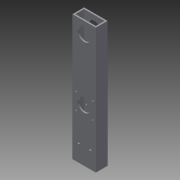
# Autodesk Inventor part: ArmSupport
Saved by Autodesk Inventor 2013 (Build 170138000, 138)
## iProperties
Created: 2014-01-22
Part Number: ArmSupport
Material: Generic
Document SubType Name: Modeling
Designer: 215152
Density: 1 g/cm^3
Author: 215152
Autodesk Inventor part; units mm, degrees
ref_plane "YZ Plane" through (0, 0, 0) normal (1, 0, 0) x (0, 1, 0)
ref_plane "XZ Plane" through (0, 0, 0) normal (0, 1, 0) x (-1, 0, 0)
ref_plane "XY Plane" through (0, 0, 0) normal (0, 0, 1) x (1, 0, 0)
sketch "Sketch1" plane through (0, 0, 0) normal (0, 1, 0) x (-1, 0, 0)
  line L0 (25.4, 12.7) -> (-25.4, 12.7)
  line L1 (-25.4, 12.7) -> (-25.4, -12.7)
  line L2 (-25.4, -12.7) -> (25.4, -12.7)
  line L3 (25.4, -12.7) -> (25.4, 12.7)
  line L4 (25.4, 12.7) -> (-25.4, -12.7) construction
  line L5 (-25.4, 12.7) -> (25.4, -12.7) construction
  line L6 (22.225, 9.525) -> (-22.225, 9.525)
  line L7 (-22.225, 9.525) -> (-22.225, -9.525)
  line L8 (-22.225, -9.525) -> (22.225, -9.525)
  line L9 (22.225, -9.525) -> (22.225, 9.525)
  line L10 (22.225, 9.525) -> (-22.225, -9.525) construction
  line L11 (-22.225, 9.525) -> (22.225, -9.525) construction
  point P0 (0, 0)
  dimension "d0" = 50.8
  dimension "d1" = 25.4
  dimension "d2" = 44.45
  dimension "d3" = 19.05
  constraints: 24 end point, 4 midpoint, 4 parallel, 2 horizontal, 2 perpendicular
  measures "d0" distance of L2.end L1.end
  measures "d1" distance of L1.end L0.end
  measures "d2" distance of L8.end L7.end
  measures "d3" distance of L7.end L6.end
extrude "Extrusion1" add sketch "Sketch1" along normal blind 273.05
sketch "Sketch2" plane through (-25.4, 0, 12.7) normal (0, 0, 1) x (1, 0, 0)
  line L0 (0, 0) -> (0, 273.05) projected
  line L1 (25.4, 0) -> (25.4, 38.1)
  line L2 (25.4, 0) -> (63.5, 0) construction
  line L3 (25.4, 38.1) -> (38.1, 38.1)
  line L4 (38.1, 38.1) -> (12.7, 38.1)
  circle A0 centre (12.7, 38.1) radius 3.175
  circle A1 centre (38.1, 38.1) radius 3.175
  dimension "d6" = 38.1
  dimension "d7" = 90
  dimension "d8" = 12.7
  dimension "d9" = 90
  dimension "d10" = 25.4
  dimension "d11" = 0
  dimension "d12" = 6.35
  dimension "d13" = 6.35
  constraints: 8 end point, 3 perpendicular, 2 centre point, 2 coincident, 1 horizontal, 1 parallel
  measures "d6" distance of L1.start L1.end
  measures "d7" angle of L2 L1
  measures "d8" distance of L1.end L3.end
  measures "d9" angle of L1 L3
  measures "d10" distance of L3.end L4.end
  measures "d11" distance between parallel lines of L4 L3
  measures "d12" diameter of A0
  measures "d13" diameter of A1
extrude "Extrusion2" cut sketch "Sketch2" against normal blind 203.2
sketch "Sketch3" plane through (-25.4, 0, 12.7) normal (0, 0, 1) x (1, 0, 0)
  line L0 (0, 273.05) -> (50.8, 273.05) projected
  line L1 (0, 0) -> (0, 273.05) projected
  line L2 (25.4, 273.05) -> (25.4, 247.65)
  line L3 (25.4, 273.05) -> (50.8, 273.05) construction
  circle A0 centre (25.4, 247.65) radius 14.2875
  point P0 (25.4, 0)
  dimension "d16" = 25.4
  dimension "d17" = 90
  dimension "d18" = 28.575
  constraints: 4 end point, 1 centre point, 1 coincident, 1 horizontal, 1 midpoint, 1 parallel, 1 perpendicular
  measures "d16" distance of L2.start L2.end
  measures "d17" angle of L2 L3
  measures "d18" diameter of A0
extrude "Extrusion3" cut sketch "Sketch3" against normal blind 25.4
sketch "Sketch4" plane through (-25.4, 0, 12.7) normal (0, 0, 1) x (1, 0, 0)
  line L0 (0, 0) -> (50.8, 0)
  line L1 (50.8, 0) -> (50.8, 76.2)
  line L2 (0, 76.2) -> (0, 0)
  line L3 (50.8, 76.2) -> (0, 76.2)
  line L4 (0, 76.2) -> (0, 127)
  line L5 (50.8, 127) -> (50.8, 76.2)
  circle A0 centre (25.4, 114.3) radius 14.2875
  line L6 (25.4, 114.3) -> (50.8, 114.3) construction
  circle A1 centre (7.4395, 132.2605) radius 2.032
  circle A2 centre (7.4395, 96.3395) radius 2.032
  circle A3 centre (43.3605, 96.3395) radius 2.032
  circle A4 centre (43.3605, 132.2605) radius 2.032
  point P0 (25.4, 0)
  dimension "d21" = 50.8
  dimension "d22" = 76.2
  dimension "d23" = 50.8
  dimension "d24" = 50.8
  dimension "d25" = 28.575
  dimension "d29" = 4.064
  dimension "d30" = 4.064
  dimension "d31" = 4.064
  dimension "d32" = 4.064
  dimension "d35" = 38.1
  dimension "d36" = 56.0605
  dimension "d37" = 56.0605
  dimension "d38" = 20.1395
  dimension "d39" = 20.1395
  constraints: 14 end point, 5 centre point, 3 horizontal, 2 parallel, 2 perpendicular
  measures "d21" distance of L2.start L1.end
  measures "d22" distance of L1.end L0.end
  measures "d23" distance of L4.end L5.start
  measures "d24" distance of L3.end L4.end
  measures "d25" diameter of A0
  measures "d29" diameter of A1
  measures "d30" diameter of A2
  measures "d31" diameter of A3
  measures "d32" diameter of A4
  measures "d35" distance from line of L3 L6.start
  measures "d36" distance from line of L3 A1.centre
  measures "d37" distance from line of L3 A4.centre
  measures "d38" distance from line of A3.centre L3
  measures "d39" distance from line of A2.centre L3
extrude "Extrusion4" cut sketch "Sketch4" against normal blind 25.4 contours A0 | A1 | A2 | A3 | A4
body "Solid1"
